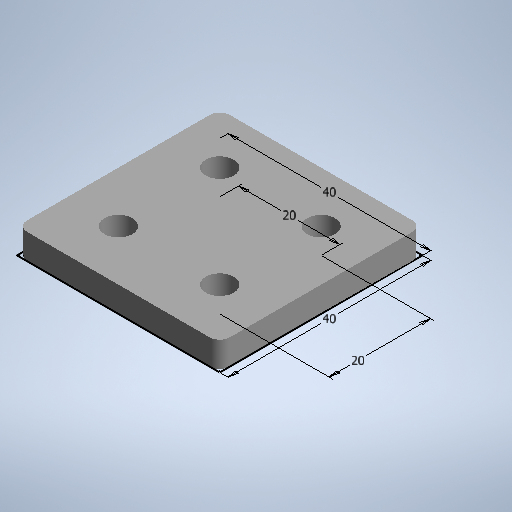
# Autodesk Inventor part: 4040Square
Saved by Autodesk Inventor 2025.4 (Build 294407000, 407)
## iProperties
Created: 2026-07-08
Part Number: 4040Square
Material: Générique
Document SubType Name: Modeling
Designer: louis
Density: 1 g/cm^3
Appearance: Par défaut
Author: louis
Autodesk Inventor part; units mm, degrees
ref_plane "YZ Plane" through (0, 0, 0) normal (1, 0, 0) x (0, 1, 0)
ref_plane "XZ Plane" through (0, 0, 0) normal (0, 1, 0) x (-1, 0, 0)
ref_plane "XY Plane" through (0, 0, 0) normal (0, 0, 1) x (1, 0, 0)
sketch "Sketch2" plane through (0, 0, 0) normal (0, 0, 1) x (1, 0, 0)
  line L0 (-20, -20) -> (20, -20)
  line L1 (20, -20) -> (20, 20)
  line L2 (20, 20) -> (-20, 20)
  line L3 (-20, 20) -> (-20, -20)
  line L4 (-20, -20) -> (20, 20) construction
  line L5 (20, -20) -> (-20, 20) construction
  line L6 (-10, -10) -> (10, -10) construction
  line L7 (10, -10) -> (10, 10) construction
  line L8 (10, 10) -> (-10, 10) construction
  line L9 (-10, 10) -> (-10, -10) construction
  line L10 (-10, -10) -> (10, 10) construction
  line L11 (10, -10) -> (-10, 10) construction
  point P0 (0, 0)
  dimension "d0" = 40
  dimension "d1" = 40
  dimension "d2" = 20
  dimension "d3" = 20
  constraints: 24 end point, 4 coincident, 4 midpoint, 4 parallel, 2 horizontal, 2 perpendicular
  measures "d0" distance of L2.end L1.end
  measures "d1" distance of L1.end L0.end
  measures "d2" distance of L8.end L7.end
  measures "d3" distance between parallel lines of L6 L8
extrude "Extrusion1" add sketch "Sketch2" along normal blind 5
hole "Hole1" at (-10, 10, 0) at (10, 10, 0) at (10, -10, 0) at (-10, -10, 0) direction (0, 0, 1) diameter 5.5 end through all clearance for "Flat Head Machine Screw" size "M5" standard "Ansi Metric M Profile"
fillet "Fillet1" radius 2 4 edges at (20, 20, 2.5) (-20, 20, 2.5) (-20, -20, 2.5) (20, -20, 2.5)
body "Solid1"
